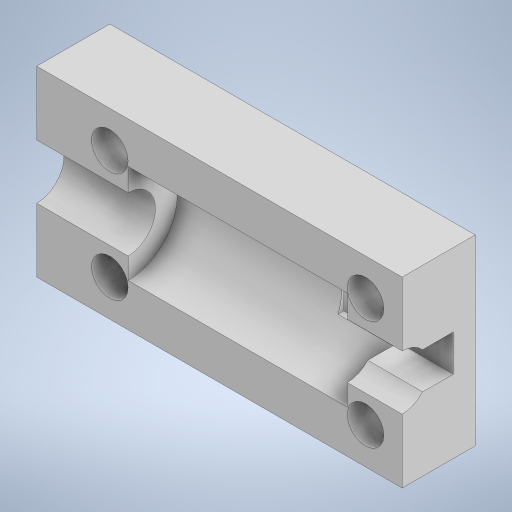
# Autodesk Inventor part: lase_top
Saved by Autodesk Inventor 2024 (Build 280153000, 153)
## iProperties
Created: 2023-11-01
Part Number: lase_top
Material: Generic
Document SubType Name: Modeling
Designer: toybox
Density: 1 g/cm^3
Appearance: Default
Author: toybox
Autodesk Inventor part; units mm, degrees
sketch "Sketch1" plane through (0, 0, 0) normal (0, 0, 1) x (1, 0, 0)
  line L0 (-10, 5) -> (10, 5)
  line L1 (10, 5) -> (10, -5)
  line L2 (10, -5) -> (-10, -5)
  line L3 (-10, -5) -> (-10, 5)
  line L4 (-10, 5) -> (10, -5) construction
  line L5 (10, 5) -> (-10, -5) construction
  point P0 (0, 0)
  dimension "d0" = 20
  dimension "d1" = 10
  constraints: 12 end point, 2 midpoint, 2 parallel, 1 horizontal, 1 perpendicular
  measures "d0" distance of L1.end L2.end
  measures "d1" distance of L0.end L1.end
extrude "Extrusion1" add sketch "Sketch1" along normal blind 4
sketch "Sketch5" plane through (10, -5, 0) normal (1, 0, 0) x (0, 0, -1)
  circle A0 centre (-4, 5) radius 1.5
  point P0 (0, 5)
  dimension "d16" = 3
  constraints: 1 centre point
  measures "d16" diameter of A0
extrude "Extrusion4" cut sketch "Sketch5" against normal through all
ref_plane "Work Plane2" through (-5, 0, -0.0356) normal (-1, 0, 0) x (0, 0, 1)
sketch "Sketch6" plane through (-5, 0, -0.0356) normal (-1, 0, 0) x (0, 0, 1)
  arc A0 (4.0356, -1.4565) -> (4.0356, 1.5435) centre (4.0356, 0.0435) ccw
  circle A1 centre (4.0356, 0.0435) radius 2.7
  point P0 (8.0356, 0.0435)
  dimension "d20" = 5.4
  constraints: 2 centre point, 2 point on circle, 1 coincident
  measures "d20" diameter of A1
extrude "Extrusion5" cut sketch "Sketch6" against normal blind 12
sketch "Sketch7" plane through (0, 0, 4) normal (0, 0, 1) x (1, 0, 0)
  circle A0 centre (8, 3) radius 1
  circle A1 centre (8, -3) radius 1
  circle A2 centre (-6, 3) radius 1
  circle A3 centre (-6, -3) radius 1
  point P0 (0, 0)
  dimension "d26" = 2
  dimension "d27" = 2
  dimension "d28" = 2
  dimension "d29" = 2
  constraints: 4 centre point
  measures "d26" diameter of A0
  measures "d27" diameter of A1
  measures "d28" diameter of A2
  measures "d29" diameter of A3
extrude "Extrusion6" cut sketch "Sketch7" against normal through all
ref_plane "Work Plane3" through (-80, 0.5, 0) normal (0, 1, 0) x (1, 0, 0)
ref_plane "Work Plane4" through (-80, 0.2, 0) normal (0, 1, 0) x (1, 0, 0)
ref_plane "Work Plane5" through (-80, 0, 0) normal (0, 1, 0) x (1, 0, 0)
sketch "Sketch10" plane through (-80, 0, 0) normal (0, 1, 0) x (1, 0, 0)
  line L0 (90, -2.5) -> (90, -4)
  line L1 (90, -4) -> (84, -4)
  line L2 (84, -4) -> (84, -1.2)
  line L3 (84, -1.2) -> (90, -1.2)
  line L4 (90, -1.2) -> (90, -4)
  point P0 (45, 0)
  dimension "d42" = 6
  dimension "d43" = 2.8
  constraints: 10 end point, 2 parallel, 1 horizontal, 1 perpendicular
  measures "d42" distance of L2.end L3.end
  measures "d43" distance of L1.end L2.end
extrude "Extrusion9" cut sketch "Sketch10" along normal mid plane 2
sketch "Sketch12" plane through (0, 0, 0) normal (0, 0, -1) x (-1, 0, 0)
  line L0 (7.6493, -1.6216) -> (-9.1144, -1.6216) construction
  line L1 (-9.1144, -1.6216) -> (-9.1144, 1.4284) construction
  line L2 (-9.1144, 1.4284) -> (7.6493, 1.4284) construction
  line L3 (7.6493, 1.4284) -> (7.6493, -1.6216) construction
  spline S0 degree 2 poles (6.7615, -1.4284) (6.7615, -1.6216) (6.5654, -1.6216) knots 0 0 0 1 1 1
  spline S1 degree 2 poles (6.5654, -1.6216) (6.3693, -1.6216) (6.3693, -1.4284) knots 0 0 0 1 1 1
  line L4 (6.3693, -1.4284) -> (6.3693, 1.039)
  line L5 (6.3693, 1.039) -> (5.3807, 1.039)
  spline S2 degree 2 poles (5.3807, 1.039) (5.1846, 1.039) (5.1846, 1.2323) knots 0 0 0 1 1 1
  spline S3 degree 2 poles (5.1846, 1.2323) (5.1846, 1.4284) (5.3807, 1.4284) knots 0 0 0 1 1 1
  line L6 (5.3807, 1.4284) -> (6.5654, 1.4284)
  spline S4 degree 2 poles (6.5654, 1.4284) (6.7615, 1.4284) (6.7615, 1.2323) knots 0 0 0 1 1 1
  line L7 (6.7615, 1.2323) -> (6.7615, -1.4284)
  spline S5 degree 2 poles (2.8012, 1.4284) (3.0729, 1.4284) (3.4426, 1.0587) (3.4426, 0.787) knots 0 0 0 1 2 2 2
  spline S6 degree 2 poles (3.4426, 0.787) (3.4426, 0.6161) (3.3558, 0.4677) knots 0 0 0 1 1 1
  spline S7 degree 2 poles (3.3558, 0.4677) (3.1765, 0.1512) (2.8012, 0.1512) knots 0 0 0 1 1 1
  line L8 (2.8012, 0.1512) -> (2.2579, 0.1512)
  line L9 (2.2579, 0.1512) -> (2.2579, -0.1008)
  spline S8 degree 2 poles (2.2579, -0.1008) (2.2579, -0.2045) (2.4007, -0.3473) (2.5071, -0.3473) knots 0 0 0 1 2 2 2
  line L10 (2.5071, -0.3473) -> (3.0981, -0.3473)
  spline S9 degree 2 poles (3.0981, -0.3473) (3.2941, -0.3473) (3.2941, -0.5434) knots 0 0 0 1 1 1
  spline S10 degree 2 poles (3.2941, -0.5434) (3.2941, -0.7366) (3.0981, -0.7366) knots 0 0 0 1 1 1
  line L11 (3.0981, -0.7366) -> (2.5071, -0.7366)
  spline S11 degree 2 poles (2.5071, -0.7366) (2.2383, -0.7366) (1.8658, -0.3669) (1.8658, -0.1008) knots 0 0 0 1 2 2 2
  line L12 (1.8658, -0.1008) -> (1.8658, 1.2323)
  spline S12 degree 2 poles (1.8658, 1.2323) (1.8658, 1.4284) (2.0618, 1.4284) knots 0 0 0 1 1 1
  line L13 (2.0618, 1.4284) -> (2.8012, 1.4284)
  line L14 (2.2579, 0.5405) -> (2.8012, 0.5405)
  spline S13 degree 2 poles (2.8012, 0.5405) (2.9048, 0.5405) (3.0505, 0.6862) (3.0505, 0.787) knots 0 0 0 1 2 2 2
  spline S14 degree 2 poles (3.0505, 0.787) (3.0505, 0.8906) (2.902, 1.039) (2.8012, 1.039) knots 0 0 0 1 2 2 2
  line L15 (2.8012, 1.039) -> (2.2579, 1.039)
  line L16 (2.2579, 1.039) -> (2.2579, 0.5405)
  spline S15 degree 2 poles (-1.0638, 0.8626) (-1.0638, 0.7506) (-0.9658, 0.703) knots 0 0 0 1 1 1
  line L17 (-0.9658, 0.703) -> (-0.2068, 0.3389)
  spline S16 degree 2 poles (-0.2068, 0.3389) (0.1181, 0.182) (0.1181, -0.1737) knots 0 0 0 1 1 1
  spline S17 degree 2 poles (0.1181, -0.1737) (0.1181, -0.4537) (-0.1144, -0.605) knots 0 0 0 1 1 1
  spline S18 degree 2 poles (-0.1144, -0.605) (-0.3076, -0.7338) (-0.5933, -0.7338) knots 0 0 0 1 1 1
  spline S19 degree 2 poles (-0.5933, -0.7338) (-0.9378, -0.7338) (-1.2066, -0.563) knots 0 0 0 1 1 1
  spline S20 degree 2 poles (-1.2066, -0.563) (-1.3075, -0.4986) (-1.3075, -0.3949) knots 0 0 0 1 1 1
  spline S21 degree 2 poles (-1.3075, -0.3949) (-1.3075, -0.3137) (-1.1926, -0.1989) (-1.1114, -0.1989) knots 0 0 0 1 2 2 2
  spline S22 degree 2 poles (-1.1114, -0.1989) (-1.0582, -0.1989) (-0.9966, -0.2409) knots 0 0 0 1 1 1
  spline S23 degree 2 poles (-0.9966, -0.2409) (-0.8173, -0.3445) (-0.5933, -0.3445) knots 0 0 0 1 1 1
  spline S24 degree 2 poles (-0.5933, -0.3445) (-0.274, -0.3445) (-0.274, -0.1737) knots 0 0 0 1 1 1
  spline S25 degree 2 poles (-0.274, -0.1737) (-0.274, -0.0588) (-0.3664, -0.014) knots 0 0 0 1 1 1
  line L18 (-0.3664, -0.014) -> (-1.1338, 0.3557)
  spline S26 degree 2 poles (-1.1338, 0.3557) (-1.4559, 0.5125) (-1.4559, 0.8626) knots 0 0 0 1 1 1
  spline S27 degree 2 poles (-1.4559, 0.8626) (-1.4559, 1.1595) (-1.2206, 1.3079) knots 0 0 0 1 1 1
  spline S28 degree 2 poles (-1.2206, 1.3079) (-1.0302, 1.4284) (-0.7277, 1.4284) knots 0 0 0 1 1 1
  spline S29 degree 2 poles (-0.7277, 1.4284) (-0.288, 1.4284) (0.0117, 1.2575) knots 0 0 0 1 1 1
  spline S30 degree 2 poles (0.0117, 1.2575) (0.1181, 1.1987) (0.1181, 1.0839) knots 0 0 0 1 1 1
  spline S31 degree 2 poles (0.1181, 1.0839) (0.1181, 1.0054) (0.0033, 0.8906) (-0.0779, 0.8906) knots 0 0 0 1 2 2 2
  spline S32 degree 2 poles (-0.0779, 0.8906) (-0.1172, 0.8906) (-0.134, 0.899) knots 0 0 0 1 1 1
  spline S33 degree 2 poles (-0.134, 0.899) (-0.2152, 0.9354) (-0.3664, 0.9886) knots 0 0 0 1 1 1
  spline S34 degree 2 poles (-0.3664, 0.9886) (-0.5485, 1.039) (-0.7361, 1.039) knots 0 0 0 1 1 1
  spline S35 degree 2 poles (-0.7361, 1.039) (-1.0638, 1.039) (-1.0638, 0.8626) knots 0 0 0 1 1 1
  line L19 (-3.5957, 0.5405) -> (-3.5957, 0.787)
  spline S36 degree 2 poles (-3.5957, 0.787) (-3.5957, 0.8906) (-3.7441, 1.039) (-3.8449, 1.039) knots 0 0 0 1 2 2 2
  line L20 (-3.8449, 1.039) -> (-4.5843, 1.039)
  spline S37 degree 2 poles (-4.5843, 1.039) (-4.7804, 1.039) (-4.7804, 1.2323) knots 0 0 0 1 1 1
  spline S38 degree 2 poles (-4.7804, 1.2323) (-4.7804, 1.4284) (-4.5843, 1.4284) knots 0 0 0 1 1 1
  line L21 (-4.5843, 1.4284) -> (-3.8449, 1.4284)
  spline S39 degree 2 poles (-3.8449, 1.4284) (-3.5733, 1.4284) (-3.2036, 1.0587) (-3.2036, 0.7898) knots 0 0 0 1 2 2 2
  line L22 (-3.2036, 0.7898) -> (-3.2036, 0.0504)
  spline S40 degree 2 poles (-3.2036, 0.0504) (-3.2036, -0.2745) (-3.6629, -0.7338) (-3.9906, -0.7338) knots 0 0 0 1 2 2 2
  spline S41 degree 2 poles (-3.9906, -0.7338) (-4.3239, -0.7338) (-4.7804, -0.2801) (-4.7804, 0.0504) knots 0 0 0 1 2 2 2
  line L23 (-4.7804, 0.0504) -> (-4.7804, 0.5405)
  line L24 (-4.7804, 0.5405) -> (-3.5957, 0.5405)
  spline S42 degree 2 poles (-3.9906, -0.3473) (-3.8281, -0.3473) (-3.5957, -0.1149) (-3.5957, 0.0476) knots 0 0 0 1 2 2 2
  line L25 (-3.5957, 0.0476) -> (-3.5957, 0.1512)
  line L26 (-3.5957, 0.1512) -> (-4.3883, 0.1512)
  line L27 (-4.3883, 0.1512) -> (-4.3883, 0.0476)
  spline S43 degree 2 poles (-4.3883, 0.0476) (-4.3883, -0.1149) (-4.1558, -0.3473) (-3.9906, -0.3473) knots 0 0 0 1 2 2 2
  spline S44 degree 2 poles (-6.6737, -0.5434) (-6.6737, -0.7366) (-6.8697, -0.7366) knots 0 0 0 1 1 1
  line L28 (-6.8697, -0.7366) -> (-7.7576, -0.7366)
  spline S45 degree 2 poles (-7.7576, -0.7366) (-7.9536, -0.7366) (-7.9536, -0.5434) knots 0 0 0 1 1 1
  line L29 (-7.9536, -0.5434) -> (-7.9536, -0.2465)
  spline S46 degree 2 poles (-7.9536, -0.2465) (-7.9536, -0.0504) (-7.7576, -0.0504) knots 0 0 0 1 1 1
  spline S47 degree 2 poles (-7.7576, -0.0504) (-7.5615, -0.0504) (-7.5615, -0.2465) knots 0 0 0 1 1 1
  line L30 (-7.5615, -0.2465) -> (-7.5615, -0.3473)
  line L31 (-7.5615, -0.3473) -> (-7.0658, -0.3473)
  line L32 (-7.0658, -0.3473) -> (-7.0658, 1.2323)
  spline S48 degree 2 poles (-7.0658, 1.2323) (-7.0658, 1.4284) (-6.8697, 1.4284) knots 0 0 0 1 1 1
  spline S49 degree 2 poles (-6.8697, 1.4284) (-6.6737, 1.4284) (-6.6737, 1.2323) knots 0 0 0 1 1 1
  line L33 (-6.6737, 1.2323) -> (-6.6737, -0.5434)
  point P0 (0, 0)
  constraints: 2 other
extrude "Extrusion10" cut sketch "Sketch12" against normal blind 0.5
body "Solid1"
